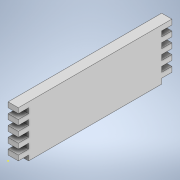
# Autodesk Inventor part: Parameter Practice
Saved by Autodesk Inventor 2022 (Build 260153000, 153)
## iProperties
Created: 2023-06-25
Part Number: Parameter Practice
Material: Generic
Document SubType Name: Modeling
Designer: Eric Cao
Density: 1 g/cm^3
Appearance: Default
Author: Eric Cao
Autodesk Inventor part; units mm, degrees
ref_plane "YZ Plane" through (0, 0, 0) normal (1, 0, 0) x (0, 1, 0)
ref_plane "XZ Plane" through (0, 0, 0) normal (0, 1, 0) x (-1, 0, 0)
ref_plane "XY Plane" through (0, 0, 0) normal (0, 0, 1) x (1, 0, 0)
sketch "Sketch1" plane through (0, 0, 0) normal (1, 0, 0) x (0, 1, 0)
  point P0 (0, 0)
sketch "Sketch2" plane through (0, 0, 0) normal (1, 0, 0) x (0, 1, 0)
  line L0 (0, 0) -> (100, 0)
  line L1 (100, 0) -> (100, -300)
  line L2 (100, -300) -> (0, -300)
  line L3 (0, -300) -> (0, 0)
  dimension "d0" = 100
  dimension "d1" = 300
  constraints: 8 end point, 2 parallel, 1 horizontal, 1 perpendicular
  measures "d0" distance of L1.end L2.end
  measures "d1" distance of L0.end L1.end
extrude "Extrusion1" add sketch "Sketch2" along normal blind 20
sketch "Sketch3" plane through (20, 0, 0) normal (1, 0, 0) x (0, 0, -1)
  line L0 (0, 0) -> (20, 0)
  line L1 (20, 0) -> (20, 10)
  line L2 (20, 10) -> (0, 10)
  line L3 (0, 0) -> (0, 10)
  line L4 (0, 100) -> (0, 0) construction
  line L5 (0, 20) -> (20, 20)
  line L6 (20, 20) -> (20, 30)
  line L7 (20, 30) -> (0, 30)
  line L8 (0, 20) -> (0, 30)
  line L9 (0, 40) -> (20, 40)
  line L10 (20, 40) -> (20, 50)
  line L11 (20, 50) -> (0, 50)
  line L12 (0, 40) -> (0, 50)
  line L13 (0, 60) -> (20, 60)
  line L14 (20, 60) -> (20, 70)
  line L15 (20, 70) -> (0, 70)
  line L16 (0, 60) -> (0, 70)
  line L17 (0, 80) -> (20, 80)
  line L18 (20, 80) -> (20, 90)
  line L19 (20, 90) -> (0, 90)
  line L20 (0, 80) -> (0, 90)
  line L21 (0, 0) -> (300, 0) construction
  line L22 (280, 0) -> (300, 0)
  line L23 (300, 0) -> (300, 10)
  line L24 (300, 10) -> (280, 10)
  line L25 (280, 0) -> (280, 10)
  line L26 (280, 20) -> (300, 20)
  line L27 (300, 20) -> (300, 30)
  line L28 (280, 20) -> (280, 30)
  line L29 (300, 30) -> (280, 30)
  line L30 (280, 40) -> (300, 40)
  line L31 (300, 40) -> (300, 50)
  line L32 (280, 40) -> (280, 50)
  line L33 (300, 50) -> (280, 50)
  line L34 (280, 60) -> (300, 60)
  line L35 (300, 60) -> (300, 70)
  line L36 (300, 70) -> (280, 70)
  line L37 (280, 80) -> (300, 80)
  line L38 (300, 80) -> (300, 90)
  line L39 (300, 90) -> (280, 90)
  line L40 (280, 80) -> (280, 90)
  line L41 (280, 60) -> (280, 70)
  dimension "d17" = 1
  dimension "d5" = 10
  dimension "d6" = 20
  dimension "d9" = 20
  dimension "d16" = 280
  dimension "d21" = 10
  constraints: 80 end point, 2 vertical, 1 horizontal, 72 other
  measures "d5" distance between parallel lines of L2 L0
  measures "d6" distance between parallel lines of L1 L3
  measures "d9" distance of L0.end L5.end
  measures "d16" distance of L0.end L22.end
  measures "d21" distance between parallel lines of L5 L2
extrude "Extrusion2" cut sketch "Sketch3" against normal blind 64.25
equation "\"d5\" = slot_width"
equation "\"d6\" = pattern_spacing"
equation "\"d9\" = pattern_spacing"
equation "\"d21\" = slot_spacing"
equation "\"slot_spacing\" = 10"
equation "\"slot_width\" = slot_spacing"
equation "\"pattern_spacing\" = 20"
body "Solid1"
